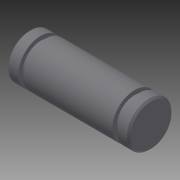
# Autodesk Inventor part: D-8383
Saved by Autodesk Inventor 2014 (Build 180170000, 170)
## iProperties
Category: PARTsolutions
Company: BIMBA
Created: 2014-01-18
Part Number: D-8383
Material: Generic
Catalog Web Link: www.cadenas.de
Description: Piston Rod Clevis for Original Line Cylinders - Pin-
Vendor: BIMBA
Document SubType Name: Standard Catalog Part
Designer: Andrew Toennies
Manufacturer: BIMBA
Density: 1 g/cm^3
Appearance: RGB(191.25000000000000,191.25000000000000,191.25000000000000)
PSOL_IDENT_0: {$CADENAS_DATA\23d-libs\bimba\bimba\bimba_imperial\bimba_full_line\original_line_cylinders\accessori
PSOL_IDENT_1: es\piston_rod_clevis_pin.prj},199 {VTYP=3D},{NB=D-8383},{LINA=D-8383},{NN=Piston Rod Clevis for Orig
PSOL_IDENT_2: inal Line Cylinders - Pin},{DATE=03.04.2013 10:23:40},{GEOMDATE=03.04.2013 12:23:00},{VERSION=},{LIN
PSOL_IDENT_3: EID=40},{LINESUBID=-1},{WBVAR=}  {NB=D-8383},{LINA=D-8383},{KT=DUMMY},{PN=D-8383},{L=1.03100000},{L1=
PSOL_IDENT_4: 0.75500000},{L2=0.04050000},{L4=0.09800000},{D=0.37650000},{D1=0.30450000},{CH=0.01500000},{R=0.0025
PSOL_IDENT_5: 0000},{COLOR=0.75,0.75,0.75,0.00}
CNS_NN: Piston Rod Clevis for Original Line Cylinders - Pin
CNS_NB: D-8383
CNS_NBSYN: $PN.
CNS_LINA: D-8383
CNS_PN: D-8383
CNS_L: 1.03100000
CNS_L1: 0.75500000
CNS_L2: 0.04050000
CNS_L4: 0.09800000
CNS_D: 0.37650000
CNS_D1: 0.30450000
CNS_CH: 0.01500000
CNS_R: 0.00250000
CNS_COLOR: 0.75,0.75,0.75,0.00
SUPPLIER: BIMBA
ARTICLENO: D-8383
BOMINFO: D-8383
CREATOR: CADENAS GmbH
Title: D-8383
Author: Cadenas PARTsolutions
Autodesk Inventor part; units mm, degrees
ref_plane "YZ Plane" through (0, 0, 0) normal (1, 0, 0) x (0, 1, 0)
ref_plane "XZ Plane" through (0, 0, 0) normal (0, 1, 0) x (-1, 0, 0)
ref_plane "XY Plane" through (0, 0, 0) normal (0, 0, 1) x (1, 0, 0)
sketch "Sketch_1" plane through (0, 0, 0) normal (0, 0, 1) x (1, 0, 0)
  line L0 (13.0937, 0) -> (-13.0937, 0)
  line L1 (-13.0937, 0) -> (-13.0937, 4.4005)
  line L2 (-13.0937, 4.4005) -> (-12.7127, 4.7816)
  line L3 (-12.7127, 4.7816) -> (-10.6172, 4.7816)
  line L4 (-10.6172, 4.7816) -> (-10.6172, 3.8671)
  line L5 (-10.6172, 3.8671) -> (-9.5885, 3.8671)
  line L6 (-9.5885, 3.8671) -> (-9.5885, 4.7816)
  line L7 (-9.5885, 4.7816) -> (9.5885, 4.7816)
  line L8 (9.5885, 4.7816) -> (9.5885, 3.8671)
  line L9 (9.5885, 3.8671) -> (10.6172, 3.8671)
  line L10 (10.6172, 3.8671) -> (10.6172, 4.7816)
  line L11 (10.6172, 4.7816) -> (12.7127, 4.7816)
  line L12 (12.7127, 4.7816) -> (13.0937, 4.4005)
  line L13 (13.0937, 4.4005) -> (13.0937, 0)
  line L14 (13.0937, 0) -> (-13.0937, 0)
  constraints: 30 end point
revolve "Revolution1" add sketch "Sketch_1" angle 360 about axis through (13.0937, 0, 0) along (1, 0, 0)
ref_plane "p1_XY" through (0, 0, 4.7816) normal (1, 0, 0) x (0, 0, -1)
ref_plane "p1_YZ" through (0, 0, 4.7816) normal (0, 0, -1) x (0, 1, 0)
ref_plane "p1_ZX" through (0, 0, 4.7816) normal (0, 1, 0) x (1, 0, 0)
ref_plane "p2_XY" through (0, 0, -4.7816) normal (1, 0, 0) x (0, 0, -1)
ref_plane "p2_YZ" through (0, 0, -4.7816) normal (0, 0, -1) x (0, 1, 0)
ref_plane "p2_ZX" through (0, 0, -4.7816) normal (0, 1, 0) x (1, 0, 0)
ref_plane "pin_XY" through (0, 0, 0) normal (1, 0, 0) x (0, 0, -1)
ref_plane "pin_YZ" through (0, 0, 0) normal (0, 0, -1) x (0, 1, 0)
ref_plane "pin_ZX" through (0, 0, 0) normal (0, 1, 0) x (1, 0, 0)
ref_plane "rr1_XY" through (10.1029, 0, 0) normal (1, 0, 0) x (0, 0, -1)
ref_plane "rr1_YZ" through (10.1029, 0, 0) normal (0, 0, -1) x (0, 1, 0)
ref_plane "rr1_ZX" through (10.1029, 0, 0) normal (0, 1, 0) x (1, 0, 0)
ref_plane "rr2_XY" through (-10.1029, 0, 0) normal (1, 0, 0) x (0, 0, -1)
ref_plane "rr2_YZ" through (-10.1029, 0, 0) normal (0, 0, -1) x (0, 1, 0)
ref_plane "rr2_ZX" through (-10.1029, 0, 0) normal (0, 1, 0) x (1, 0, 0)
ref_plane "w21_XY" through (13.0937, 0, 0) normal (0, 1, 0) x (1, 0, 0)
ref_plane "w21_YZ" through (13.0937, 0, 0) normal (1, 0, 0) x (0, 0, -1)
ref_plane "w21_ZX" through (13.0937, 0, 0) normal (0, 0, -1) x (0, 1, 0)
ref_plane "w22_XY" through (-13.0937, 0, 0) normal (0, 1, 0) x (1, 0, 0)
ref_plane "w22_YZ" through (-13.0937, 0, 0) normal (1, 0, 0) x (0, 0, -1)
ref_plane "w22_ZX" through (-13.0937, 0, 0) normal (0, 0, -1) x (0, 1, 0)
body "Solid1"
